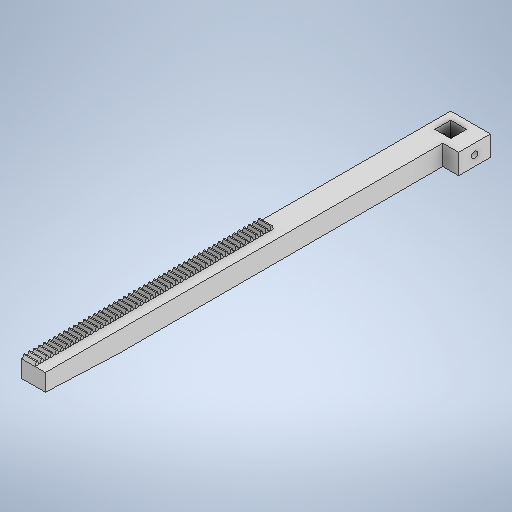
# Autodesk Inventor part: cremaillere
Saved by Autodesk Inventor 2025.2 (Build 292293000, 293)
## iProperties
Created: 2025-03-30
Part Number: cremaillere
Material: Générique
Document SubType Name: Modeling
Designer: enezl
Density: 1 g/cm^3
Appearance: Par défaut
Author: enezl
Autodesk Inventor part; units mm, degrees
ref_plane "YZ Plane" through (0, 0, 0) normal (1, 0, 0) x (0, 1, 0)
ref_plane "XZ Plane" through (0, 0, 0) normal (0, 1, 0) x (-1, 0, 0)
ref_plane "XY Plane" through (0, 0, 0) normal (0, 0, 1) x (1, 0, 0)
sketch "dent" plane through (0, 0, 0) normal (0, 0, 1) x (1, 0, 0)
  line L0 (3.4049, 12.8641) -> (5.6549, 12.0451)
  line L1 (5.6549, 12.0451) -> (5.6549, 11.2941)
  line L2 (5.6549, 11.2941) -> (3.4049, 10.4751)
  line L3 (3.4049, 10.4751) -> (3.4049, 9.7241)
  point P0 (4.4433, 11.2784)
  dimension "d0" = 2.25
  dimension "d1" = 110
  dimension "d2" = 40
  dimension "d3" = 3.14
  measures "d3" distance of point (3.405, 9.724) point (3.405, 12.864)
sketch "Esquisse1" plane through (0, 0, 0) normal (1, 0, 0) x (0, 1, 0)
  line L0 (12.75, 135) -> (12.75, -15) construction
  line L1 (12.75, 135) -> (2, 135)
  line L2 (0, 135) -> (0, -135) construction
  line L3 (0, -135) -> (12.75, -135)
  line L4 (12.75, -15.72) -> (12.75, -135)
  line L5 (2, 135) -> (0, 89.1925)
  line L6 (2, 135) -> (0, 135) construction
  line L7 (0, 89.1925) -> (0, -135)
  line L8 (12.75, 135) -> (15, 134.1811)
  line L9 (15, 134.1811) -> (15, 133.43)
  line L10 (15, 133.43) -> (12.75, 132.6111)
  line L11 (12.75, 132.6111) -> (12.75, 131.86)
  line L12 (12.75, 131.86) -> (15, 131.0411)
  line L13 (15, 131.0411) -> (15, 130.29)
  line L14 (15, 130.29) -> (12.75, 129.4711)
  line L15 (12.75, 129.4711) -> (12.75, 128.72)
  line L16 (12.75, 128.72) -> (15, 127.9011)
  line L17 (15, 127.9011) -> (15, 127.15)
  line L18 (15, 127.15) -> (12.75, 126.3311)
  line L19 (12.75, 126.3311) -> (12.75, 125.58)
  line L20 (12.75, 125.58) -> (15, 124.7611)
  line L21 (15, 124.7611) -> (15, 124.01)
  line L22 (15, 124.01) -> (12.75, 123.1911)
  line L23 (12.75, 123.1911) -> (12.75, 122.44)
  line L24 (12.75, 122.44) -> (15, 121.6211)
  line L25 (15, 121.6211) -> (15, 120.87)
  line L26 (15, 120.87) -> (12.75, 120.0511)
  line L27 (12.75, 120.0511) -> (12.75, 119.3)
  line L28 (12.75, 119.3) -> (15, 118.4811)
  line L29 (15, 118.4811) -> (15, 117.73)
  line L30 (15, 117.73) -> (12.75, 116.9111)
  line L31 (12.75, 116.9111) -> (12.75, 116.16)
  line L32 (12.75, 116.16) -> (15, 115.3411)
  line L33 (15, 115.3411) -> (15, 114.59)
  line L34 (15, 114.59) -> (12.75, 113.7711)
  line L35 (12.75, 113.7711) -> (12.75, 113.02)
  line L36 (12.75, 113.02) -> (15, 112.2011)
  line L37 (15, 112.2011) -> (15, 111.45)
  line L38 (15, 111.45) -> (12.75, 110.6311)
  line L39 (12.75, 110.6311) -> (12.75, 109.88)
  line L40 (12.75, 109.88) -> (15, 109.0611)
  line L41 (15, 109.0611) -> (15, 108.31)
  line L42 (15, 108.31) -> (12.75, 107.4911)
  line L43 (12.75, 107.4911) -> (12.75, 106.74)
  line L44 (12.75, 106.74) -> (15, 105.9211)
  line L45 (15, 105.9211) -> (15, 105.17)
  line L46 (15, 105.17) -> (12.75, 104.3511)
  line L47 (12.75, 104.3511) -> (12.75, 103.6)
  line L48 (12.75, 103.6) -> (15, 102.7811)
  line L49 (15, 102.7811) -> (15, 102.03)
  line L50 (15, 102.03) -> (12.75, 101.2111)
  line L51 (12.75, 101.2111) -> (12.75, 100.46)
  line L52 (12.75, 100.46) -> (15, 99.6411)
  line L53 (15, 99.6411) -> (15, 98.89)
  line L54 (15, 98.89) -> (12.75, 98.0711)
  line L55 (12.75, 98.0711) -> (12.75, 97.32)
  line L56 (12.75, 97.32) -> (15, 96.5011)
  line L57 (15, 96.5011) -> (15, 95.75)
  line L58 (15, 95.75) -> (12.75, 94.9311)
  line L59 (12.75, 94.9311) -> (12.75, 94.18)
  line L60 (12.75, 94.18) -> (15, 93.3611)
  line L61 (15, 93.3611) -> (15, 92.61)
  line L62 (15, 92.61) -> (12.75, 91.7911)
  line L63 (12.75, 91.7911) -> (12.75, 91.04)
  line L64 (12.75, 91.04) -> (15, 90.2211)
  line L65 (15, 90.2211) -> (15, 89.47)
  line L66 (15, 89.47) -> (12.75, 88.6511)
  line L67 (12.75, 88.6511) -> (12.75, 87.9)
  line L68 (12.75, 87.9) -> (15, 87.0811)
  line L69 (15, 87.0811) -> (15, 86.33)
  line L70 (15, 86.33) -> (12.75, 85.5111)
  line L71 (12.75, 85.5111) -> (12.75, 84.76)
  line L72 (12.75, 84.76) -> (15, 83.9411)
  line L73 (15, 83.9411) -> (15, 83.19)
  line L74 (15, 83.19) -> (12.75, 82.3711)
  line L75 (12.75, 82.3711) -> (12.75, 81.62)
  line L76 (12.75, 81.62) -> (15, 80.8011)
  line L77 (15, 80.8011) -> (15, 80.05)
  line L78 (15, 80.05) -> (12.75, 79.2311)
  line L79 (12.75, 79.2311) -> (12.75, 78.48)
  line L80 (12.75, 78.48) -> (15, 77.6611)
  line L81 (15, 77.6611) -> (15, 76.91)
  line L82 (15, 76.91) -> (12.75, 76.0911)
  line L83 (12.75, 76.0911) -> (12.75, 75.34)
  line L84 (12.75, 75.34) -> (15, 74.5211)
  line L85 (15, 74.5211) -> (15, 73.77)
  line L86 (15, 73.77) -> (12.75, 72.9511)
  line L87 (12.75, 72.9511) -> (12.75, 72.2)
  line L88 (12.75, 72.2) -> (15, 71.3811)
  line L89 (15, 71.3811) -> (15, 70.63)
  line L90 (15, 70.63) -> (12.75, 69.8111)
  line L91 (12.75, 69.8111) -> (12.75, 69.06)
  line L92 (12.75, 69.06) -> (15, 68.2411)
  line L93 (15, 68.2411) -> (15, 67.49)
  line L94 (15, 67.49) -> (12.75, 66.6711)
  line L95 (12.75, 66.6711) -> (12.75, 65.92)
  line L96 (12.75, 65.92) -> (15, 65.1011)
  line L97 (15, 65.1011) -> (15, 64.35)
  line L98 (15, 64.35) -> (12.75, 63.5311)
  line L99 (12.75, 63.5311) -> (12.75, 62.78)
  line L100 (12.75, 62.78) -> (15, 61.9611)
  line L101 (15, 61.9611) -> (15, 61.21)
  line L102 (15, 61.21) -> (12.75, 60.3911)
  line L103 (12.75, 60.3911) -> (12.75, 59.64)
  line L104 (12.75, 59.64) -> (15, 58.8211)
  line L105 (15, 58.8211) -> (15, 58.07)
  line L106 (15, 58.07) -> (12.75, 57.2511)
  line L107 (12.75, 57.2511) -> (12.75, 56.5)
  line L108 (12.75, 56.5) -> (15, 55.6811)
  line L109 (15, 55.6811) -> (15, 54.93)
  line L110 (15, 54.93) -> (12.75, 54.1111)
  line L111 (12.75, 54.1111) -> (12.75, 53.36)
  line L112 (12.75, 53.36) -> (15, 52.5411)
  line L113 (15, 52.5411) -> (15, 51.79)
  line L114 (15, 51.79) -> (12.75, 50.9711)
  line L115 (12.75, 50.9711) -> (12.75, 50.22)
  line L116 (12.75, 50.22) -> (15, 49.4011)
  line L117 (15, 49.4011) -> (15, 48.65)
  line L118 (15, 48.65) -> (12.75, 47.8311)
  line L119 (12.75, 47.8311) -> (12.75, 47.08)
  line L120 (12.75, 47.08) -> (15, 46.2611)
  line L121 (15, 46.2611) -> (15, 45.51)
  line L122 (15, 45.51) -> (12.75, 44.6911)
  line L123 (12.75, 44.6911) -> (12.75, 43.94)
  line L124 (12.75, 43.94) -> (15, 43.1211)
  line L125 (15, 43.1211) -> (15, 42.37)
  line L126 (15, 42.37) -> (12.75, 41.5511)
  line L127 (12.75, 41.5511) -> (12.75, 40.8)
  line L128 (12.75, 40.8) -> (15, 39.9811)
  line L129 (15, 39.9811) -> (15, 39.23)
  line L130 (15, 39.23) -> (12.75, 38.4111)
  line L131 (12.75, 38.4111) -> (12.75, 37.66)
  line L132 (12.75, 37.66) -> (15, 36.8411)
  line L133 (15, 36.8411) -> (15, 36.09)
  line L134 (15, 36.09) -> (12.75, 35.2711)
  line L135 (12.75, 35.2711) -> (12.75, 34.52)
  line L136 (12.75, 34.52) -> (15, 33.7011)
  line L137 (15, 33.7011) -> (15, 32.95)
  line L138 (15, 32.95) -> (12.75, 32.1311)
  line L139 (12.75, 32.1311) -> (12.75, 31.38)
  line L140 (12.75, 31.38) -> (15, 30.5611)
  line L141 (15, 30.5611) -> (15, 29.81)
  line L142 (15, 29.81) -> (12.75, 28.9911)
  line L143 (12.75, 28.9911) -> (12.75, 28.24)
  line L144 (12.75, 28.24) -> (15, 27.4211)
  line L145 (15, 27.4211) -> (15, 26.67)
  line L146 (15, 26.67) -> (12.75, 25.8511)
  line L147 (12.75, 25.8511) -> (12.75, 25.1)
  line L148 (12.75, 25.1) -> (15, 24.2811)
  line L149 (15, 24.2811) -> (15, 23.53)
  line L150 (15, 23.53) -> (12.75, 22.7111)
  line L151 (12.75, 22.7111) -> (12.75, 21.96)
  line L152 (12.75, 21.96) -> (15, 21.1411)
  line L153 (15, 21.1411) -> (15, 20.39)
  line L154 (15, 20.39) -> (12.75, 19.5711)
  line L155 (12.75, 19.5711) -> (12.75, 18.82)
  line L156 (12.75, 18.82) -> (15, 18.0011)
  line L157 (15, 18.0011) -> (15, 17.25)
  line L158 (15, 17.25) -> (12.75, 16.4311)
  line L159 (12.75, 16.4311) -> (12.75, 15.68)
  line L160 (12.75, 15.68) -> (15, 14.8611)
  line L161 (15, 14.8611) -> (15, 14.11)
  line L162 (15, 14.11) -> (12.75, 13.2911)
  line L163 (12.75, 13.2911) -> (12.75, 12.54)
  line L164 (12.75, 12.54) -> (15, 11.7211)
  line L165 (15, 11.7211) -> (15, 10.97)
  line L166 (15, 10.97) -> (12.75, 10.1511)
  line L167 (12.75, 10.1511) -> (12.75, 9.4)
  line L168 (12.75, 9.4) -> (15, 8.5811)
  line L169 (15, 8.5811) -> (15, 7.83)
  line L170 (15, 7.83) -> (12.75, 7.0111)
  line L171 (12.75, 7.0111) -> (12.75, 6.26)
  line L172 (12.75, 6.26) -> (15, 5.4411)
  line L173 (15, 5.4411) -> (15, 4.69)
  line L174 (15, 4.69) -> (12.75, 3.8711)
  line L175 (12.75, 3.8711) -> (12.75, 3.12)
  line L176 (12.75, 3.12) -> (15, 2.3011)
  line L177 (15, 2.3011) -> (15, 1.55)
  line L178 (15, 1.55) -> (12.75, 0.7311)
  line L179 (12.75, 0.7311) -> (12.75, -0.02)
  line L180 (12.75, -0.02) -> (15, -0.8389)
  line L181 (15, -0.8389) -> (15, -1.59)
  line L182 (15, -1.59) -> (12.75, -2.4089)
  line L183 (12.75, -2.4089) -> (12.75, -3.16)
  line L184 (12.75, -3.16) -> (15, -3.9789)
  line L185 (15, -3.9789) -> (15, -4.73)
  line L186 (15, -4.73) -> (12.75, -5.5489)
  line L187 (12.75, -5.5489) -> (12.75, -6.3)
  line L188 (12.75, -6.3) -> (15, -7.1189)
  line L189 (15, -7.1189) -> (15, -7.87)
  line L190 (15, -7.87) -> (12.75, -8.6889)
  line L191 (12.75, -8.6889) -> (12.75, -9.44)
  line L192 (12.75, -9.44) -> (15, -10.2589)
  line L193 (15, -10.2589) -> (15, -11.01)
  line L194 (15, -11.01) -> (12.75, -11.8289)
  line L195 (12.75, -11.8289) -> (12.75, -12.58)
  line L196 (12.75, -12.58) -> (15, -13.3989)
  line L197 (15, -13.3989) -> (15, -14.15)
  line L198 (15, -14.15) -> (12.75, -14.9689)
  line L199 (12.75, -14.9689) -> (12.75, -15.72)
  point P0 (0, 0)
  point P1 (0, 0)
  point P2 (12.75, -12.58)
  point P3 (12.75, -6.3)
  point P4 (12.75, -3.16)
  point P5 (12.75, -0.02)
  point P6 (12.75, 3.12)
  point P7 (12.75, 9.4)
  point P8 (12.75, 18.82)
  point P9 (12.75, 21.96)
  point P10 (12.75, 25.1)
  point P11 (12.75, 28.24)
  point P12 (12.75, 31.38)
  point P13 (12.75, 34.52)
  point P14 (12.75, 37.66)
  point P15 (12.75, 40.8)
  point P16 (12.75, 47.08)
  point P17 (12.75, 50.22)
  point P18 (12.75, 53.36)
  point P19 (12.75, 56.5)
  point P20 (12.75, 59.64)
  point P21 (12.75, 62.78)
  point P22 (12.75, 65.92)
  point P23 (12.75, 69.06)
  point P24 (12.75, 81.62)
  point P25 (12.75, 84.76)
  point P26 (12.75, 87.9)
  point P27 (12.75, 91.04)
  point P28 (12.75, 94.18)
  point P29 (12.75, 106.74)
  point P30 (12.75, 113.02)
  point P31 (12.75, 119.3)
  point P32 (12.75, 125.58)
  point P33 (12.75, 131.86)
  dimension "d7" = 3.14
  dimension "d4" = 150
  dimension "d12" = 15
  dimension "d13" = 270
  dimension "d14" = 2.5
  dimension "d15" = 2
  constraints: 50 vertical, 16 end point, 3 perpendicular, 2 horizontal, 1 coincident, 1 collinear, 1 midpoint, 1 point on line, 2 other
  measures "d4" distance of L0.start L0.end
  measures "d13" distance of L2.start L2.end
  measures "d14" angle of L2 L5
  measures "d15" distance of L1.end L2.start
extrude "Extrusion1" add sketch "Esquisse1" along normal blind 8
sketch "Esquisse2" plane through (8, 0, 0) normal (1, 0, 0) x (0, 0, -1)
  line L0 (-135, 2) -> (-89.1925, 0) projected
  line L1 (-135, 12.75) -> (-135, 2) projected
  line L2 (135, 12.75) -> (14.9689, 12.75) projected
  line L3 (-89.1925, 0) -> (135, 0) projected
  line L4 (135, 0) -> (135, 12.75) projected
  line L5 (-135, 12.75) -> (14.9689, 12.75)
  point P0 (0, 0)
  constraints: 2 end point, 1 collinear
extrude "Extrusion2" add sketch "Esquisse2" along normal blind 6.5 and the other way blind 8.5
sketch "Esquisse3" plane through (14.5, 0, 0) normal (1, 0, 0) x (0, 0, -1)
  line L0 (135, 0) -> (-89.1925, 0) construction
  line L1 (-135, 12.75) -> (135, 12.75) construction
  line L2 (135, 0) -> (115, 0)
  line L3 (115, 0) -> (115, 12.75)
  line L4 (115, 12.75) -> (135, 12.75)
  line L5 (135, 12.75) -> (135, 0)
  line L6 (125, 12.75) -> (125, 0) construction
  point P0 (0, 0)
  point P1 (125, 6.375)
  point P2 (125, 6.375)
  point P3 (125, 6.375)
  dimension "d22" = 20
  constraints: 10 end point, 3 midpoint, 2 coincident, 2 parallel, 1 horizontal, 1 perpendicular, 1 point on line
  measures "d22" distance between parallel lines of L5 L3
extrude "Extrusion3" add sketch "Esquisse3" along normal blind 10
hole "Perçage1" at (14.5, 6.375, -125) direction (-1, 0, 0) diameter 3.2 end through all start extended yes counterbore diameter 4 counterbore depth 2
sketch "Esquisse4" plane through (0, 12.75, 132.6111) normal (0, 1, 0) x (1, 0, 0)
  line L0 (14.5, 252.6111) -> (4.5, 252.6111)
  line L1 (4.5, 252.6111) -> (4.5, 262.6111)
  line L2 (4.5, 262.6111) -> (14.5, 262.6111)
  line L3 (14.5, 262.6111) -> (14.5, 252.6111)
  line L4 (14.5, 252.6111) -> (4.5, 262.6111) construction
  line L5 (4.5, 252.6111) -> (14.5, 262.6111) construction
  line L6 (24.5, 247.6111) -> (24.5, 267.6111) construction
  line L7 (24.5, 257.6111) -> (-0.5, 257.6111) construction
  line L8 (-0.5, 256.0111) -> (-0.5, 259.2111) construction
  line L9 (-0.5, -2.3889) -> (-0.5, 267.6111) construction
  point P0 (0, 132.6111)
  point P1 (9.5, 257.6111)
  dimension "d32" = 10
  dimension "d33" = 10
  dimension "d34" = 5
  constraints: 14 end point, 4 midpoint, 2 parallel, 1 horizontal, 1 perpendicular, 1 point on line
  measures "d32" distance of L0.end L1.end
  measures "d33" distance of L1.end L2.end
  measures "d34" distance between parallel lines of L9 L1
extrude "Extrusion4" cut sketch "Esquisse4" against normal through all
